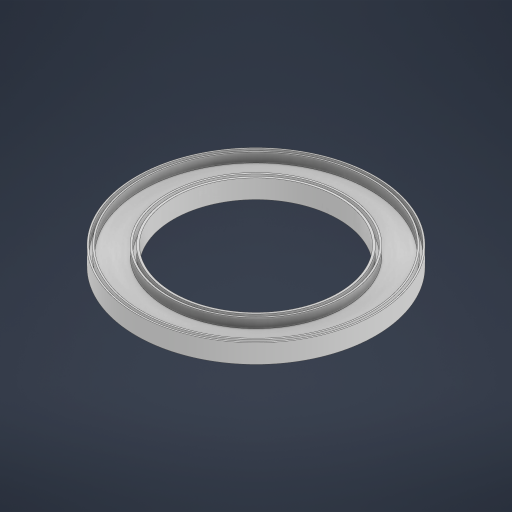
# Autodesk Inventor part: PethFormaFlanec
Saved by Autodesk Inventor 2024 (Build 280153000, 153)
## iProperties
Created: 2023-12-11
Part Number: PethFormaFlanec
Material: Generic
Document SubType Name: Modeling
Designer: KirikDK
Mass: 160.499 g
Surface Area: 774.065 cm^2
Volume: 160.499 cm^3
Density: 1 g/cm^3
Appearance: Default
Author: KirikDK
Autodesk Inventor part; units mm, degrees
ref_plane "YZ Plane" through (0, 0, 0) normal (1, 0, 0) x (0, 1, 0)
ref_plane "XZ Plane" through (0, 0, 0) normal (0, 1, 0) x (-1, 0, 0)
ref_plane "XY Plane" through (0, 0, 0) normal (0, 0, 1) x (1, 0, 0)
sketch "Sketch1" plane through (0, 0, 0) normal (0, 1, 0) x (-1, 0, 0)
  circle A0 centre (0.143, 11.2846) radius 71.8694
  circle A1 centre (0.143, 11.2846) radius 74.247
  circle A2 centre (0.143, 11.2846) radius 98.333
  circle A3 centre (0.143, 11.2846) radius 100.5055
  circle A4 centre (0.143, 11.2846) radius 70.1276
  circle A5 centre (0.143, 11.2846) radius 75.7155
  circle A6 centre (0.143, 11.2846) radius 97.0759
  circle A7 centre (0.143, 11.2846) radius 101.7155
  point P0 (0, 0)
  constraints: 8 centre point, 7 coincident
extrude "Extrusion1" add sketch "Sketch1" along normal blind 8
sketch "Sketch2" plane through (-0.143, 0, 11.2846) normal (0, -1, 0) x (1, 0, 0)
  circle A0 centre (0, 0) radius 101.7155
  circle A1 centre (0, 0) radius 70.1276
  point P0 (0.143, -11.2846)
  constraints: 2 centre point, 1 coincident
extrude "Extrusion2" add sketch "Sketch2" along normal blind 8
body "Solid1"
